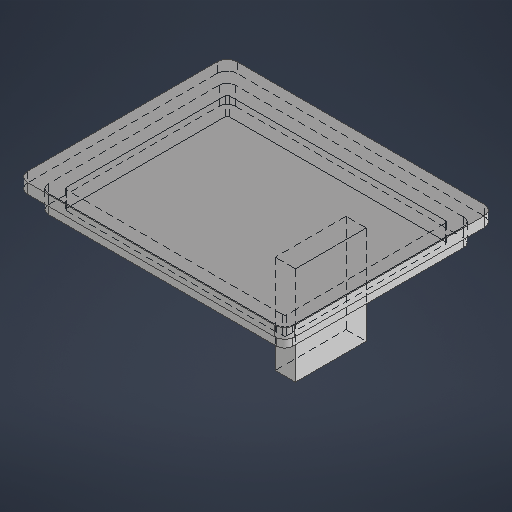
# Autodesk Inventor part: kucisteGornji
Saved by Autodesk Inventor 2025.2 (Build 292293000, 293)
## iProperties
Created: 2024-12-18
Part Number: kucisteGornji
Material: Generic
Document SubType Name: Modeling
Designer: antem
Density: 1 g/cm^3
Appearance: Default
Author: antem
Autodesk Inventor part; units mm, degrees
ref_plane "YZ Plane" through (0, 0, 0) normal (1, 0, 0) x (0, 1, 0)
ref_plane "XZ Plane" through (0, 0, 0) normal (0, 1, 0) x (-1, 0, 0)
ref_plane "XY Plane" through (0, 0, 0) normal (0, 0, 1) x (1, 0, 0)
sketch "Sketch1" plane through (0, 0, 0) normal (0, 0, 1) x (1, 0, 0)
  line L0 (-66, 51.75) -> (66, 51.75)
  line L1 (66, 51.75) -> (66, -51.75)
  line L2 (66, -51.75) -> (-66, -51.75)
  line L3 (-66, -51.75) -> (-66, 51.75)
  line L4 (-60.5, 46.25) -> (60.5, 46.25)
  line L5 (60.5, 46.25) -> (60.5, -46.25)
  line L6 (60.5, -46.25) -> (-60.5, -46.25)
  line L7 (-60.5, -46.25) -> (-60.5, 46.25)
  line L8 (54.5, 40.25) -> (-54.5, 40.25)
  line L9 (-54.5, 40.25) -> (-54.5, -40.25)
  line L10 (-54.5, -40.25) -> (54.5, -40.25)
  line L11 (54.5, -40.25) -> (54.5, 40.25)
  line L12 (0, 46.25) -> (0, 40.25) construction
  line L13 (-60.5, 0) -> (-54.5, 0) construction
  line L14 (0, 51.75) -> (0, 46.25) construction
  line L15 (-60.5, 0) -> (-66, 0) construction
  line L16 (37, 17.5) -> (27, 17.5)
  line L17 (27, 17.5) -> (27, -17.5)
  line L18 (27, -17.5) -> (37, -17.5)
  line L19 (37, -17.5) -> (37, 17.5)
  line L20 (66, -46.75) -> (66, 46.75)
  line L21 (-61, -51.75) -> (61, -51.75)
  line L22 (-61, 46.75) -> (61, 46.75)
  line L23 (61, 46.75) -> (61, -46.75)
  point P0 (0, 0)
  point P1 (60.5, 0)
  point P2 (66, 0)
  point P3 (37, 0)
  point P4 (54.5, 0)
  dimension "d9" = 0.5
  dimension "d10" = 6
  dimension "d11" = 10
  dimension "d12" = 35
  dimension "d13" = 24
  constraints: 48 end point, 10 midpoint, 8 parallel, 7 perpendicular, 6 horizontal, 4 horizontal alignment, 4 vertical, 3 vertical alignment, 2 collinear, 7 other
  measures "d9" distance between parallel lines of L23 L5
  measures "d10" distance between parallel lines of L11 L5
  measures "d11" distance of L17.end L18.end
  measures "d12" distance of L18.end L16.start
  measures "d13" distance between parallel lines of L23 L19
extrude "Extrusion1" add sketch "Sketch1" along normal blind 5 contours L0 L1 L2 L3 | L4 L5 L6 L7 | L11 L10 L9 L8 | L19 L18 L17 L16
extrude "Extrusion2" add sketch "Sketch1" against normal blind 9 contours L4 L5 L6 L7
extrude "Extrusion3" add sketch "Sketch1" against normal blind 48.5 contours L19 L18 L17 L16
fillet "Fillet1" radius 5 4 edges at (66, 51.75, 2.5) (-66, 51.75, 2.5) (66, -51.75, 2.5) (-66, -51.75, 2.5)
fillet "Fillet2" radius 4 4 edges at (-60.5, -46.25, -4.5) (60.5, -46.25, -4.5) (60.5, 46.25, -4.5) (-60.5, 46.25, -4.5)
fillet "Fillet3" radius 1 4 edges at (54.5, -40.25, -4.5) (-54.5, -40.25, -4.5) (54.5, 40.25, -4.5) (-54.5, 40.25, -4.5)
body "Solid1"
